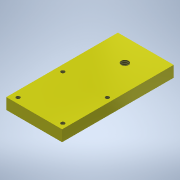
# Autodesk Inventor part: mirror translation stage adapter v2
Saved by Autodesk Inventor 2022 (Build 260153000, 153)
## iProperties
Created: 2009-10-27
Part Number: mirror translation stage adapter v2
Document SubType Name: Modeling
Designer: betzige
Density: 1 g/cm^3
Material: Generic
Appearance: Smooth - Yellow
Author: betzige
Autodesk Inventor part; units mm, degrees
ref_plane "YZ Plane" through (0, 0, 0) normal (1, 0, 0) x (0, 1, 0)
ref_plane "XZ Plane" through (0, 0, 0) normal (0, 1, 0) x (-1, 0, 0)
ref_plane "XY Plane" through (0, 0, 0) normal (0, 0, 1) x (1, 0, 0)
sketch "Sketch1" plane through (0, 0, 0) normal (0, 0, 1) x (1, 0, 0)
  line L0 (0, 0) -> (25, 0)
  line L1 (25, 0) -> (25, 50)
  line L2 (25, 50) -> (0, 50)
  line L3 (0, 50) -> (0, 0)
  dimension "d0" = 50
  dimension "d1" = 25
  constraints: 8 end point, 2 parallel, 1 horizontal, 1 perpendicular
  measures "d0" distance of L0.end L1.end
  measures "d1" distance of L0.start L0.end
extrude "Extrusion1" add sketch "Sketch1" along normal blind 5
sketch "Sketch7" plane through (0, 0, 0) normal (0, 0, -1) x (-1, 0, 0)
  line L0 (0, 0) -> (-25, 0) projected
  line L1 (0, 50) -> (0, 0) projected
  line L2 (-25, 50) -> (0, 50) projected
  line L3 (-25, 0) -> (-25, 50) projected
  line L4 (-26.9321, 31.3954) -> (-26.9317, 31.395) projected
  line L5 (-6.036, 52.1675) -> (-6.0379, 52.1694) projected
  line L6 (-6.0392, 52.1707) -> (-6.0403, 52.1719) projected
  line L7 (-25, 50) -> (-17.5538, 50)
  line L8 (-9.8347, 48.3993) -> (-9.8243, 48.3993)
  line L9 (-25, 50) -> (-25, 43.2194)
  line L10 (-25, 33.3181) -> (-25, 33.3148)
  line L11 (-25, 50) -> (-25, 0)
  line L12 (-25, 0) -> (0, 0)
  line L13 (0, 0) -> (0, 50)
  line L14 (-4.3266, 37.6341) -> (0, 42.0051)
  line L15 (-7.4462, 50) -> (-12.072, 45.3663)
  line L16 (-12.072, 45.3663) -> (-4.3266, 37.6341)
  line L17 (-12.072, 45.3663) -> (-4.3266, 37.6341)
  point P0 (0, 33.3148)
  point P1 (0, 45.3321)
  point P2 (0, 37.6341)
  point P3 (-16.7135, 50)
  point P4 (0, 42.0051)
  dimension "d59" = 16.7135
  dimension "d60" = 7.4462
  constraints: 23 end point, 5 perpendicular, 5 point on line, 4 collinear
  measures "d59" distance of L1.start point (-16.713, 50)
  measures "d60" distance of L1.start L15.start
extrude "Extrusion3" add sketch "Sketch7" along normal blind 2 from surface at 0 contours L14 L16 L15 L2 L1
sketch "Sketch11" plane through (0, 0, 0) normal (0, 0, -1) x (-1, 0, 0)
  circle A0 centre (-13.3, 39.8488) radius 1.651
  line L0 (-25, 50) -> (-7.4462, 50) projected
  line L1 (-25, 0) -> (-25, 50) projected
  point P0 (0, 0)
  dimension "d61" = 3.302
  dimension "d62" = 10.1512
  dimension "d63" = 11.7
  constraints: 1 centre point
  measures "d61" diameter of A0
  measures "d62" distance from line of L0 A0.centre
  measures "d63" distance from line of A0.centre L1
hole "Hole5" at (13.3, 39.8488, 0) direction (0, 0, 1) diameter 3.302 end through all thread size "8-32 UNC" class "2B" standard "ANSI Unified Screw Threads"
sketch "Sketch12" plane through (0, 0, 0) normal (0, 0, -1) x (-1, 0, 0)
  circle A0 centre (-22.8048, 22.5) radius 0.847
  line L0 (0, 0) -> (-25, 0) projected
  line L1 (-25, 0) -> (-25, 50) projected
  circle A1 centre (-22.8048, 2.5) radius 0.847
  circle A2 centre (-2.8048, 22.5) radius 0.847
  line L2 (0, 42.0051) -> (0, 0) projected
  circle A3 centre (-2.8048, 2.5) radius 0.847
  dimension "d71" = 1.694
  dimension "d72" = 22.5
  dimension "d73" = 2.1952
  dimension "d74" = 1.694
  dimension "d75" = 20
  dimension "d76" = 2.8048
  dimension "d77" = 1.694
  dimension "d78" = 1.694
  constraints: 4 centre point
  measures "d71" diameter of A0
  measures "d72" distance from line of L0 A0.centre
  measures "d73" distance from line of L1 A0.centre
  measures "d74" diameter of A1
  measures "d75" distance of A1.centre A0.centre
  measures "d76" distance from line of L2 A2.centre
  measures "d77" diameter of A2
  measures "d78" diameter of A3
hole "Hole8" at (22.8048, 22.5, 0) at (22.8048, 2.5, 0) at (2.8048, 22.5, 0) at (2.8048, 2.5, 0) direction (0, 0, 1) diameter 1.6942 end through all thread size "2-56 UNC" class "2B" standard "ANSI Unified Screw Threads"
body "Solid1"
